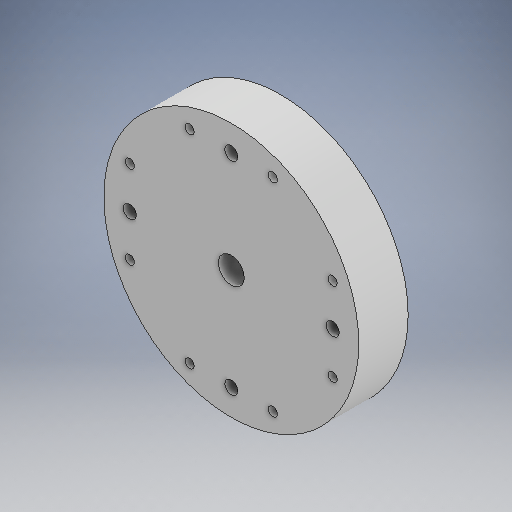
# Autodesk Inventor part: Base_Junta
Saved by Autodesk Inventor 2025.2 (Build 292293000, 293)
## iProperties
Created: 2025-04-02
Part Number: Base_Junta
Material: Generic
Document SubType Name: Modeling
Designer: Tiago
Density: 1 g/cm^3
Appearance: Default
Author: Tiago
Autodesk Inventor part; units mm, degrees
ref_plane "YZ Plane" through (0, 0, 0) normal (1, 0, 0) x (0, 1, 0)
ref_plane "XZ Plane" through (0, 0, 0) normal (0, 1, 0) x (-1, 0, 0)
ref_plane "XY Plane" through (0, 0, 0) normal (0, 0, 1) x (1, 0, 0)
sketch "Sketch1" plane through (0, 0, 0) normal (0, 0, 1) x (1, 0, 0)
  circle A0 centre (0, 0) radius 49
  circle A1 centre (0, 0) radius 5
  line L0 (0, 0) -> (0, 39) construction
  circle A2 centre (0, 39) radius 2.5
  line L1 (-16, 39) -> (16, 39) construction
  circle A3 centre (16, 39) radius 1.75
  circle A4 centre (-16, 39) radius 1.75
  circle A5 centre (-39, 16) radius 1.75
  circle A6 centre (-39, 0) radius 2.5
  circle A7 centre (-39, -16) radius 1.75
  circle A8 centre (-16, -39) radius 1.75
  circle A9 centre (0, -39) radius 2.5
  circle A10 centre (16, -39) radius 1.75
  circle A11 centre (39, -16) radius 1.75
  circle A12 centre (39, 0) radius 2.5
  circle A13 centre (39, 16) radius 1.75
  dimension "D" = 98
  dimension "d4" = 10
  dimension "d5" = 39
  dimension "d6" = 5
  dimension "d16" = 32
  dimension "d17" = 3.5
  dimension "d18" = 3.5
  dimension "d21" = 360
  constraints: 14 centre point, 5 coincident, 4 end point, 1 horizontal, 1 midpoint, 1 vertical, 25 other
  measures "D" diameter of A0
  measures "d4" diameter of A1
  measures "d5" distance of L0.start L0.end
  measures "d6" diameter of A2
  measures "d16" distance of L1.start L1.end
  measures "d17" diameter of A3
  measures "d18" diameter of A4
extrude "Extrusion1" add sketch "Sketch1" along normal blind 19 contours A0 | A2 | A3 | A4 | A5 | A6 | A7 | A8 | A9 | A10 | A11 | A12 | A13
extrude "Extrusion2" cut sketch "Sketch1" along normal up to surface (19 mm away) contours A2 | A3 | A4 | A5 | A6 | A7 | A8 | A9 | A10 | A11 | A12 | A13
body "Solid1"
